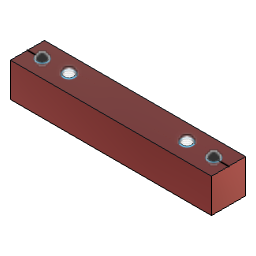
XLRTEMAssmeblyv1 (Autodesk Fusion 360 archive; units mm, degrees)
design "LoadCellSchem"
Autodesk Fusion 360 part; units mm, degrees
sketch "Sketch1" plane through (0, 0, 0) normal (0, 0, 1) x (1, 0, 0)
  line L0 (0, 0) -> (75, 0)
  line L1 (75, 0) -> (75, 12.7)
  line L2 (75, 12.7) -> (0, 12.7)
  line L3 (0, 12.7) -> (0, 0)
  dimension "d1" = 75
  dimension "d2" = 12.7
  constraint horizontal L0
  constraint vertical L1
  constraint horizontal L2
  constraint vertical L3
  constraint coincident L0.start L3.end
  measures "d1" distance of L0.start L0.end
  measures "d2" distance of L0.start L2.end
extrude "Extrude1" add sketch "Sketch1" along normal blind 12.7
sketch "Sketch2" plane through (0, 0, 12.7) normal (0, 0, 1) x (-1, 0, 0)
  line L0 (0, -12.7) -> (0, 0)
  line L1 (0, 0) -> (-75, 0)
  line L2 (-75, 0) -> (-75, -12.7)
  line L3 (-75, -12.7) -> (0, -12.7)
  circle A0 centre (-5.5, -6.35) radius 2
  circle A1 centre (-15.5, -6.35) radius 2
  circle A2 centre (-69.5, -6.35) radius 2
  circle A3 centre (-59.5, -6.35) radius 2
  line L4 (-5.5, -6.35) -> (0, -6.35)
  line L5 (-69.5, -6.35) -> (-75, -6.35)
  dimension "d5" = 4
  dimension "d6" = 4
  dimension "d7" = 10
  dimension "d8" = 4
  dimension "d9" = 4
  dimension "d10" = 10
  dimension "d11" = 44
  dimension "d12" = 64
  constraint coincident A0.centre L4.start
  constraint midpoint L0 L4.end
  constraint perpendicular L0 L4
  constraint coincident A2.centre L5.start
  constraint midpoint L2 L5.end
  constraint perpendicular L2 L5
  constraint equal L4 L5
  measures "d5" diameter of A0
  measures "d6" diameter of A1
  measures "d7" distance of A0.centre A1.centre
  measures "d8" diameter of A3
  measures "d9" diameter of A2
  measures "d10" distance of A3.centre A2.centre
  measures "d11" distance of A1.centre A3.centre
  measures "d12" distance of A0.centre A2.centre
extrude "Extrude2" cut sketch "Sketch2" against normal blind 17.78 contours A0 | A1 | A2 | A3
thread "Thread1" "ISO Metric profile 4.0 M4x0.7 6H" major diameter 4.1095 minor diameter 3.332 pitch 0.7 angle 60 resizes the face on face at (70.8965, 7.7817, 8.4667) on face at (57.5099, 6.5492, 4.2333) on face at (13.5099, 6.5491, 4.2333) on face at (3.5099, 6.5491, 4.2333)
